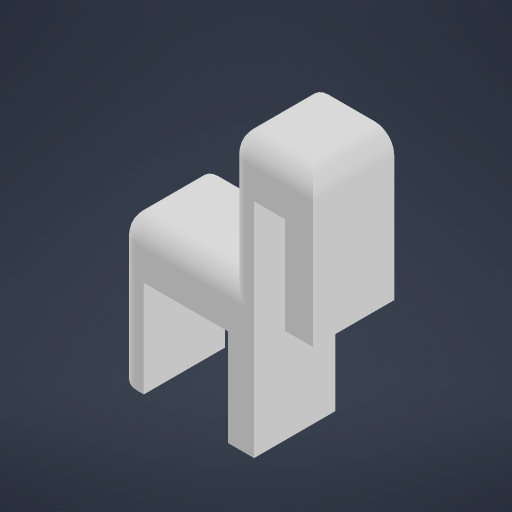
# Autodesk Inventor part: Hook_TestFit
Saved by Autodesk Inventor 2024.1 (Build 281209000, 209)
## iProperties
Created: 2023-07-11
Part Number: Hook_TestFit
Material: Generic
Document SubType Name: Modeling
Designer: User
Density: 1 g/cm^3
Appearance: Default
Author: User
Autodesk Inventor part; units mm, degrees
ref_plane "YZ Plane" through (0, 0, 0) normal (1, 0, 0) x (0, 1, 0)
ref_plane "XZ Plane" through (0, 0, 0) normal (0, 1, 0) x (-1, 0, 0)
ref_plane "XY Plane" through (0, 0, 0) normal (0, 0, 1) x (1, 0, 0)
sketch "Sketch1" plane through (0, 0, 0) normal (0, 0, 1) x (1, 0, 0)
  line L0 (0, 0) -> (-8.7, 0)
  line L1 (-8.7, 0) -> (-8.7, 8.7)
  line L2 (-8.7, 8.7) -> (0, 8.7)
  line L3 (0, 8.7) -> (0, 0)
  dimension "d0" = 8.7
  dimension "d1" = 8.7
  constraints: 8 end point, 2 parallel, 1 horizontal, 1 perpendicular
  measures "d0" distance of L1.end L2.end
  measures "d1" distance of L0.end L1.end
extrude "Extrusion1" [suppressed]
sketch "Sketch2" plane through (-8.7, 0, 0) normal (-1, 0, 0) x (0, 0, 1)
  line L0 (0, 8.7) -> (0, 0) projected
  line L1 (0, 0) -> (3, 0)
  line L2 (3, 0) -> (3, 8.7)
  line L3 (3, 8.7) -> (0, 8.7)
  line L4 (0, 8.7) -> (0, 0)
  constraints: 8 end point, 2 parallel, 1 horizontal, 1 perpendicular
extrude "Extrusion2" [suppressed]
sketch "Sketch3" plane through (0, 0, 3) normal (0, 0, 1) x (1, 0, 0)
  line L0 (0, 8.7) -> (-11.7, 8.7) projected
  line L1 (0, 0) -> (-11.7, 0) projected
  line L2 (-11.7, 8.7) -> (-8.7, 8.7)
  line L3 (-8.7, 8.7) -> (-8.7, 0)
  line L4 (-8.7, 0) -> (-11.7, 0)
  line L5 (-11.7, 0) -> (-11.7, 8.7)
  dimension "d6" = 3
  constraints: 8 end point, 2 parallel, 1 horizontal, 1 perpendicular, 1 point on line
  measures "d6" distance of L3.end L4.end
extrude "Extrusion3" [suppressed]
sketch "Sketch5" plane through (0, 0, 0) normal (1, 0, 0) x (0, 0, -1)
  line L0 (0, 8.7) -> (-3, 8.7) projected
  line L1 (0, 0) -> (-3, 0)
  line L2 (-3, 0) -> (-3, 8.7)
  line L3 (-3, 8.7) -> (0, 8.7)
  line L4 (0, 8.7) -> (0, 0)
  dimension "d9" = 3
  constraints: 8 end point, 2 parallel, 1 horizontal, 1 perpendicular
  measures "d9" distance of L0.end L3.end
extrude "Extrusion4" [suppressed]
sketch "Sketch6" plane through (0, 0, 3) normal (0, 0, 1) x (1, 0, 0)
  line L0 (3, 8.7) -> (-11.7, 8.7) projected
  line L1 (3, 8.7) -> (0, 8.7)
  line L2 (0, 8.7) -> (0, 0)
  line L3 (0, 0) -> (3, 0)
  line L4 (3, 0) -> (3, 8.7)
  constraints: 8 end point, 2 parallel, 1 horizontal, 1 perpendicular
extrude "Extrusion5" [suppressed]
sketch "Sketch7" plane through (0, 0, 0) normal (0, 0, 1) x (1, 0, 0)
  line L0 (0, 0) -> (-2.7, 0)
  line L1 (-2.7, 0) -> (-2.7, 15)
  line L2 (-2.7, 15) -> (0, 15)
  line L3 (0, 15) -> (0, 0)
  line L4 (-2.7, 15) -> (-11.4, 15)
  line L5 (-11.4, 15) -> (-11.4, 10)
  line L6 (-11.4, 10) -> (-2.7, 10)
  line L7 (-2.7, 10) -> (-2.7, 15)
  line L8 (-11.4, 15) -> (-14.1, 15)
  line L9 (-14.1, 15) -> (-14.1, 0)
  line L10 (-14.1, 0) -> (-11.4, 0)
  line L11 (-11.4, 0) -> (-11.4, 15)
  line L12 (-2.7, 15) -> (0, 15)
  line L13 (0, 15) -> (0, 23)
  line L14 (0, 23) -> (-2.7, 23)
  line L15 (-2.7, 23) -> (-2.7, 15)
  line L16 (-2.7, 23) -> (0, 23)
  line L17 (0, 23) -> (0, 28)
  line L18 (0, 28) -> (-2.7, 28)
  line L19 (-2.7, 28) -> (-2.7, 23)
  line L20 (0, 28) -> (3.2, 28)
  line L21 (3.2, 28) -> (3.2, 23)
  line L22 (3.2, 23) -> (0, 23)
  line L23 (0, 23) -> (0, 28)
  line L24 (3.2, 28) -> (6.1, 28)
  line L25 (6.1, 28) -> (6.1, 23)
  line L26 (6.1, 23) -> (3.2, 23)
  line L27 (3.2, 23) -> (3.2, 28)
  line L28 (6.1, 23) -> (3.2, 23)
  line L29 (3.2, 23) -> (3.2, 13)
  line L30 (3.2, 13) -> (6.1, 13)
  line L31 (6.1, 13) -> (6.1, 23)
  point P0 (-11.4, 10)
  point P1 (-2.7, 10)
  dimension "d14" = 2.7
  dimension "d15" = 15
  dimension "d16" = 8.7
  dimension "d17" = 5
  dimension "d18" = 2.7
  dimension "d19" = 15
  dimension "d23" = 2.7
  dimension "d24" = 8
  dimension "d25" = 5
  dimension "d26" = 3.2
  dimension "d27" = 5
  dimension "d28" = 2.9
  dimension "d29" = 2.9
  dimension "d30" = 10
  constraints: 64 end point, 16 parallel, 8 horizontal, 8 perpendicular, 1 point on line
  measures "d14" distance of L1.end L2.end
  measures "d15" distance of L0.end L1.end
  measures "d16" distance of L6.end L5.end
  measures "d17" distance of L5.end L4.end
  measures "d18" distance of L10.end L9.end
  measures "d19" distance of L9.end L8.end
  measures "d23" distance of L14.end L13.end
  measures "d24" distance of L13.end L12.end
  measures "d25" distance of L17.end L16.end
  measures "d26" distance of L21.end L22.end
  measures "d27" distance of L20.end L21.end
  measures "d28" distance of L25.end L26.end
  measures "d29" distance of L30.end L29.end
  measures "d30" distance of L29.end L28.end
extrude "Extrusion6" add sketch "Sketch7" along normal blind 8.4
fillet "Fillet1" radius 2 3 edges at (-14.1, 7.5, 8.4) (-8.4, 15, 8.4) (-14.1, 15, 4.2)
fillet "Fillet2" radius 2 4 edges at (-2.7, 21.5, 8.4) (1.7, 28, 8.4) (6.1, 28, 4.2) (-2.7, 28, 4.2)
body "Solid1"
